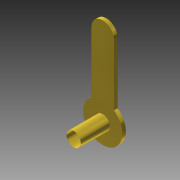
# Autodesk Inventor part: Conector
Saved by Autodesk Inventor 2013 (Build 170138000, 138)
## iProperties
Created: 2013-06-25
Part Number: Conector
Material: Genérico
Document SubType Name: Modeling
Designer: usuario
Density: 1 g/cm^3
Author: usuario
Autodesk Inventor part; units mm, degrees
ref_plane "YZ Plane" through (0, 0, 0) normal (1, 0, 0) x (0, 1, 0)
ref_plane "XZ Plane" through (0, 0, 0) normal (0, 1, 0) x (-1, 0, 0)
ref_plane "XY Plane" through (0, 0, 0) normal (0, 0, 1) x (1, 0, 0)
sketch "Boceto1" plane through (0, 0, 0) normal (0, 1, 0) x (-1, 0, 0)
  circle A0 centre (0, 0) radius 0.99
  dimension "d0" = 1.98
  constraints: 1 centre point, 1 coincident
  measures "d0" diameter of A0
extrude "Extrusión1" add sketch "Boceto1" along normal mid plane 4
sketch "Boceto2" plane through (0, 2, 0) normal (0, 1, 0) x (1, 0, 0)
  circle A0 centre (0, 0) radius 0.99 projected
  circle A1 centre (0, 0) radius 2.7
  dimension "d3" = 5.4
  constraints: 1 centre point, 1 coincident
  measures "d3" diameter of A1
extrude "Extrusión2" add sketch "Boceto2" along normal blind 0.5 contours A0 | A1
hole "Hole1" at (0, 2.5, 0) direction (0, -1, 0) diameter 1.96 end through all
hole "Hole2" at (0, 2.5, 0) direction (0, -1, 0) diameter 1.96 end through all countersink diameter 5.4 countersink angle 150
sketch "Boceto3" plane through (0, 2, 0) normal (0, -1, 0) x (1, 0, 0)
  line L0 (-1.55, 2.1185) -> (1.55, 2.1185)
  line L1 (1.55, 2.1185) -> (1.55, 10.6185)
  line L2 (1.55, 10.6185) -> (-1.55, 10.6185)
  line L3 (-1.55, 10.6185) -> (-1.55, 2.1185)
  line L4 (-1.55, 2.1185) -> (1.55, 10.6185) construction
  line L5 (1.55, 2.1185) -> (-1.55, 10.6185) construction
  point P0 (0, 6.3685)
  dimension "d24" = 3.1
  dimension "d25" = 8.5
  constraints: 12 end point, 2 midpoint, 2 parallel, 1 horizontal, 1 perpendicular
  measures "d24" distance of L2.end L1.end
  measures "d25" distance of L1.end L0.end
extrude "Extrusión3" add sketch "Boceto3" against normal blind 0.5
hole "Hole3" at (0, 2.5, 0) direction (0, -1, 0) diameter 1.96 end through all countersink diameter 5.4 countersink angle 150
sketch "Boceto4" plane through (0, 2.5, 0) normal (0, 1, 0) x (1, 0, 0)
  line L0 (-1.55, -10.6185) -> (1.55, -10.6185) projected
  circle A0 centre (0, -10.6185) radius 1.55
  dimension "d39" = 3.1
  constraints: 1 centre point, 1 midpoint
  measures "d39" diameter of A0
extrude "Extrusión4" add sketch "Boceto4" against normal blind 0.5
